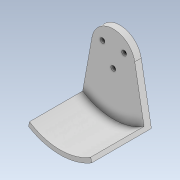
# Autodesk Inventor part: thigh_hip_connector
Saved by Autodesk Inventor 2020 (Build 240168000, 168)
## iProperties
Created: 2021-01-06
Part Number: thigh_hip_connector
Material: Generic
Document SubType Name: Modeling
Designer: DELL
Density: 1 g/cm^3
Appearance: Clear - Blue
Author: DELL
Autodesk Inventor part; units mm, degrees
ref_plane "YZ Plane" through (0, 0, 0) normal (1, 0, 0) x (0, 1, 0)
ref_plane "XZ Plane" through (0, 0, 0) normal (0, 1, 0) x (-1, 0, 0)
ref_plane "XY Plane" through (0, 0, 0) normal (0, 0, 1) x (1, 0, 0)
sketch "Sketch1" plane through (0, 0, 0) normal (0, 0, 1) x (1, 0, 0)
  circle A0 centre (0, 0) radius 20
  line L0 (-19.68, 3.5636) -> (-29, -47.9062)
  line L1 (19.68, 3.5636) -> (29, -47.9062)
  line L2 (9.9593, -5.75) -> (0, 0) construction
  circle A1 centre (8.4134, -4.8575) radius 2.5
  line L3 (0, 0) -> (9.9593, 5.75) construction
  line L4 (0, 0) -> (-9.9593, -5.75) construction
  circle A2 centre (-8.4134, -4.8575) radius 2.5
  circle A3 centre (0, 0) radius 9.715 construction
  circle A4 centre (0, 0) radius 11.5 construction
  circle A5 centre (0, 9.715) radius 2.5
  line L5 (0, 0) -> (-9.9593, 5.75) construction
  line L6 (11.5, 0) -> (-11.5, 0) construction
  circle A6 centre (-9.9593, 5.75) radius 4
  circle A7 centre (-9.9593, 5.75) radius 2.25
  line L7 (0, -48.5721) -> (0, 22.5) construction
  circle A8 centre (0, -11.5) radius 2.25
  circle A9 centre (0, -11.5) radius 4
  circle A10 centre (9.9593, 5.75) radius 4
  circle A11 centre (9.9593, 5.75) radius 2.25
  arc A12 (-28.2326, -43.6683) -> (28.2326, -43.6683) centre (0, 0) ccw
  arc A13 (-29, -47.9062) -> (29, -47.9062) centre (0, 0) ccw
  line L8 (8, -59.5) -> (-8, -59.5)
  line L9 (-8, -59.5) -> (-8, -52.5)
  line L10 (-8, -52.5) -> (8, -52.5)
  line L11 (8, -52.5) -> (8, -59.5)
  line L12 (8, -59.5) -> (-8, -52.5) construction
  line L13 (-8, -59.5) -> (8, -52.5) construction
  point P0 (0, 11.4686)
  point P1 (0, 11.4686)
  point P2 (11.5, 0)
  point P3 (-11.5, 0)
  point P4 (0, -56)
  dimension "d18" = 23
  dimension "d0" = 40
  dimension "d17" = 19.43
  dimension "d19" = 30
  dimension "d20" = 30
  dimension "d21" = 4.5
  dimension "d22" = 8
  dimension "d23" = 5
  dimension "d24" = 104
  dimension "d25" = 112
  dimension "d48" = 58
  dimension "d60" = 16
  dimension "d61" = 7
  dimension "d40" = 14
  dimension "d41" = 50
  dimension "d50" = 25
  dimension "d51" = 35
  dimension "d52" = 2.5
  dimension "d53" = 4
  constraints: 26 end point, 13 centre point, 10 coincident, 10 point on circle, 8 point on line, 6 equal radius, 2 midpoint, 2 parallel, 2 tangent, 1 horizontal, 1 perpendicular, 1 vertical, 17 other
  measures "d0" diameter of A0
  measures "d17" diameter of A3
  measures "d19" angle to the sketch x axis of L5
  measures "d20" angle to the sketch x axis of L4
  measures "d21" diameter of A11
  measures "d22" diameter of A10
  measures "d23" diameter of A5
  measures "d24" diameter of A12
  measures "d25" diameter of A13
  measures "d48" distance of L1.end L0.end
  measures "d60" distance of L8.start L8.end
  measures "d61" distance of L8.end L9.end
extrude "Extrusion1" add sketch "Sketch1" along normal blind 6 contours A0 | A0 L1 A12 L0 | L1 A13 L11 L10 L9 L0 A12 | A13 L9 L10 L11 | A1 | A2 | A5 | A6 | A9 | A10
extrude "Extrusion2" cut sketch "Sketch1" along normal blind 3.5 contours A6 | A9 | A10 | A11
extrude "Extrusion4" add sketch "Sketch1" along normal blind 49 from surface at 6 contours L1 A13 L11 L10 L9 L0 A12 | A13 L9 L10 L11
body "Solid1"
